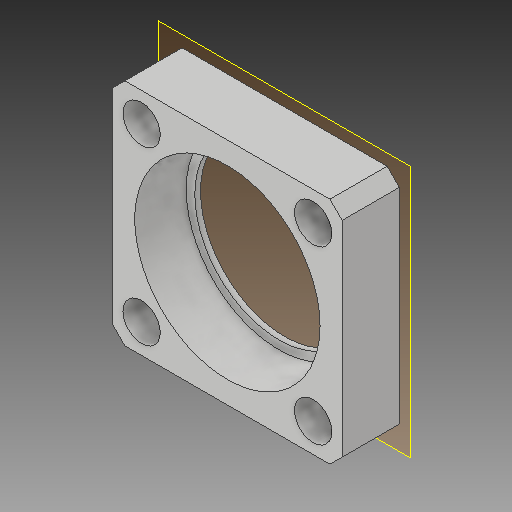
# Autodesk Inventor part: 11_Lens_Thorlabs_Mount_Customized_B
Saved by Autodesk Inventor 2019 (Build 230136000, 136)
## iProperties
Created: 2018-10-08
Part Number: 11_Lens_Thorlabs_Mount_Customized_B
Material: Generic
Document SubType Name: Modeling
Designer: diederichbenedict
Density: 1 g/cm^3
Appearance: Default
d9: 32,400 mm
Author: diederichbenedict
Autodesk Inventor part; units mm, degrees
ref_plane "YZ Plane" through (0, 0, 0) normal (1, 0, 0) x (0, 1, 0)
ref_plane "XZ Plane" through (0, 0, 0) normal (0, 1, 0) x (-1, 0, 0)
ref_plane "XY Plane" through (0, 0, 0) normal (0, 0, 1) x (1, 0, 0)
ref_plane "Work Plane1" through (0, 0, 5) normal (0, 0, 1) x (1, 0, 0)
sketch "Sketch1" plane through (0, 0, 5) normal (0, 0, 1) x (1, 0, 0)
  circle A0 centre (15, 59.8454) radius 3.2639 projected
  line L0 (-20.066, 62.7742) -> (-20.066, 26.9166)
  line L1 (-20.066, 26.9166) -> (-17.9288, 24.7794)
  line L2 (-17.9288, 24.7794) -> (17.9288, 24.7794)
  line L3 (17.9288, 24.7794) -> (20.066, 26.9166)
  line L4 (20.066, 26.9166) -> (20.066, 62.7742)
  line L5 (20.066, 62.7742) -> (17.9288, 64.9114)
  line L6 (17.9288, 64.9114) -> (-17.9288, 64.9114)
  line L7 (-17.9288, 64.9114) -> (-20.066, 62.7742)
  circle A1 centre (15, 29.8455) radius 3.2639
  circle A2 centre (15, 59.8454) radius 3.2639
  circle A3 centre (-15, 59.8454) radius 3.2639
  circle A4 centre (-15, 29.8455) radius 3.2639
  circle A5 centre (0, 44.8454) radius 16.2
  circle A6 centre (0, 44.8454) radius 12.9 construction
  point P0 (0, 0)
  dimension "d5" = 40.132
  dimension "d6" = 40.132
  dimension "d7" = 5.066
  dimension "d8" = 5.066
  dimension "d9" = 32.4
  constraints: 16 end point, 5 centre point
  measures "d5" distance between parallel lines of L2 L6
  measures "d6" distance between parallel lines of L0 L4
  measures "d7" distance from line of L4 A0.centre
  measures "d8" distance from line of L4 A1.centre
  measures "d9" diameter of A5
extrude "Extrusion1" add sketch "Sketch1" along normal blind 10
sketch "Sketch2" plane through (0, 0, 5) normal (0, 0, -1) x (-1, 0, 0)
  circle A0 centre (0, 44.8454) radius 16.2 projected
  circle A1 centre (15, 29.8455) radius 3.2639 projected
  circle A2 centre (15, 59.8454) radius 3.2639 projected
  circle A3 centre (-15, 29.8455) radius 3.2639 projected
  circle A4 centre (-15, 59.8454) radius 3.2639 projected
  line L0 (20.066, 62.7742) -> (20.066, 26.9166) projected
  line L1 (20.066, 26.9166) -> (17.9288, 24.7794) projected
  line L2 (17.9288, 24.7794) -> (-17.9288, 24.7794) projected
  line L3 (-17.9288, 24.7794) -> (-20.066, 26.9166) projected
  line L4 (-20.066, 26.9166) -> (-20.066, 62.7742) projected
  line L5 (-20.066, 62.7742) -> (-17.9288, 64.9114) projected
  line L6 (-17.9288, 64.9114) -> (17.9288, 64.9114) projected
  line L7 (17.9288, 64.9114) -> (20.066, 62.7742) projected
  circle A5 centre (0, 44.8454) radius 14.7
  point P0 (0, 0)
  dimension "d11" = 1.5
  constraints: 1 centre point
  measures "d11" radial gap between concentric circles of A0 A5
extrude "Extrusion2" add sketch "Sketch2" against normal blind 1 contours A0
body "Solid1"
